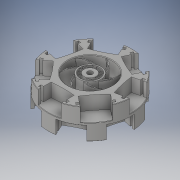
# Autodesk Inventor part: Mecanum Hub
Saved by Autodesk Inventor 2018 (Build 220112000, 112)
## iProperties
Created: 2018-03-28
Part Number: Mecanum Hub
Material: Generic
Document SubType Name: Modeling
Designer: Ajith Thomas
Density: 1 g/cm^3
Appearance: Default
Author: Ajith Thomas
Autodesk Inventor part; units mm, degrees
ref_plane "YZ Plane" through (0, 0, 0) normal (1, 0, 0) x (0, 1, 0)
ref_plane "XZ Plane" through (0, 0, 0) normal (0, 1, 0) x (-1, 0, 0)
ref_plane "XY Plane" through (0, 0, 0) normal (0, 0, 1) x (1, 0, 0)
sketch "Sketch1" plane through (0, 0, 0) normal (0, 1, 0) x (-1, 0, 0)
  circle A0 centre (0, 0) radius 18.5
  circle A1 centre (0, 0) radius 17
  dimension "d0" = 37
  dimension "d1" = 34
  constraints: 2 centre point, 2 coincident
  measures "d0" diameter of A0
  measures "d1" diameter of A1
extrude "Extrusion1" add sketch "Sketch1" along normal mid plane 23
sketch "Sketch2" plane through (0, 11.5, 0) normal (0, 1, 0) x (1, 0, 0)
  circle A0 centre (0, 0) radius 4.75
  circle A1 centre (0, 0) radius 2
  dimension "d4" = 9.5
  dimension "d5" = 4
  constraints: 2 centre point, 2 coincident
  measures "d4" diameter of A0
  measures "d5" diameter of A1
extrude "Extrusion2" add sketch "Sketch2" against normal blind 23
sketch "Sketch3" plane through (0, 0, 0) normal (0, 1, 0) x (-1, 0, 0)
  circle A0 centre (0, 0) radius 17 construction
  circle A1 centre (0, 0) radius 4.75 construction
  line L0 (12.1062, 11.9349) -> (16.389, -4.5168) construction
  arc A2 (4.7443, -0.2334) -> (12.1062, 11.9349) centre (2.5017, 9.4346) ccw
  arc A3 (2.2794, -4.1674) -> (12.1062, 11.9349) centre (0.83, 7.7668) ccw
  arc A4 (2.5742, 3.992) -> (-4.2828, 16.4517) centre (-6.9197, 6.8838) ccw
  arc A5 (4.7487, -0.1097) -> (-4.2828, 16.4517) centre (-6.3112, 4.6022) ccw
  arc A6 (-2.17, 4.2253) -> (-16.389, 4.5168) centre (-9.4214, -2.5508) ccw
  arc A7 (2.4694, 4.0577) -> (-16.389, 4.5168) centre (-7.1412, -3.1645) ccw
  arc A8 (-4.7443, 0.2334) -> (-12.1062, -11.9349) centre (-2.5017, -9.4346) ccw
  arc A9 (-2.2794, 4.1674) -> (-12.1062, -11.9349) centre (-0.83, -7.7668) ccw
  arc A10 (-2.5742, -3.992) -> (4.2828, -16.4517) centre (6.9197, -6.8838) ccw
  arc A11 (-4.7487, 0.1097) -> (4.2828, -16.4517) centre (6.3112, -4.6022) ccw
  arc A12 (2.17, -4.2253) -> (16.389, -4.5168) centre (9.4214, 2.5508) ccw
  arc A13 (-2.4694, -4.0577) -> (16.389, -4.5168) centre (7.1412, 3.1645) ccw
  arc A14 (2.2794, -4.1674) -> (4.7443, -0.2334) centre (0, 0) ccw
  arc A15 (-2.4694, -4.0577) -> (2.17, -4.2253) centre (0, 0) ccw
  arc A16 (-4.7487, 0.1097) -> (-2.5742, -3.992) centre (0, 0) ccw
  arc A17 (-2.2794, 4.1674) -> (-4.7443, 0.2334) centre (0, 0) ccw
  arc A18 (2.4694, 4.0577) -> (-2.17, 4.2253) centre (0, 0) ccw
  arc A19 (4.7487, -0.1097) -> (2.5742, 3.992) centre (0, 0) ccw
  dimension "d8" = 17
  dimension "d11" = 360
  constraints: 42 point on circle, 18 centre point, 6 concentric, 2 end point, 1 tangent, 43 other
  measures "d8" distance of L0.start L0.end
extrude "Extrusion3" add sketch "Sketch3" along normal mid plane 22
sketch "Sketch4" plane through (0, 11, 0) normal (0, 1, 0) x (1, 0, 0)
  circle A0 centre (0, 0) radius 4.75 projected
  arc A1 (-4.7443, 0.2334) -> (-12.1062, -11.9349) centre (-2.5017, -9.4346) ccw projected
  arc A2 (-2.2794, 4.1674) -> (-12.1062, -11.9349) centre (-0.83, -7.7668) ccw projected
  arc A3 (-4.6916, 0.7427) -> (-12.1429, -5.508) centre (-2.5017, -9.4346) ccw
  arc A4 (-3.1813, 3.5273) -> (-12.1429, -5.508) centre (-0.83, -7.7668) ccw
  arc A5 (-3.1813, 3.5273) -> (-4.6916, 0.7427) centre (0, 0) ccw
  arc A6 (-2.989, -3.6917) -> (-1.3014, -13.2701) centre (6.9197, -6.8838) ccw
  arc A7 (-4.6454, -0.9914) -> (-1.3014, -13.2701) centre (6.3112, -4.6022) ccw
  arc A8 (-4.6454, -0.9914) -> (-2.989, -3.6917) centre (0, 0) ccw
  arc A9 (1.7026, -4.4344) -> (10.8415, -7.7621) centre (9.4214, 2.5508) ccw
  arc A10 (-1.4641, -4.5187) -> (10.8415, -7.7621) centre (7.1412, 3.1645) ccw
  arc A11 (-1.4641, -4.5187) -> (1.7026, -4.4344) centre (0, 0) ccw
  arc A12 (4.6916, -0.7427) -> (12.1429, 5.508) centre (2.5017, 9.4346) ccw
  arc A13 (3.1813, -3.5273) -> (12.1429, 5.508) centre (0.83, 7.7668) ccw
  arc A14 (3.1813, -3.5273) -> (4.6916, -0.7427) centre (0, 0) ccw
  arc A15 (2.989, 3.6917) -> (1.3014, 13.2701) centre (-6.9197, 6.8838) ccw
  arc A16 (4.6454, 0.9914) -> (1.3014, 13.2701) centre (-6.3112, 4.6022) ccw
  arc A17 (4.6454, 0.9914) -> (2.989, 3.6917) centre (0, 0) ccw
  arc A18 (-1.7026, 4.4344) -> (-10.8415, 7.7621) centre (-9.4214, -2.5508) ccw
  arc A19 (1.4641, 4.5187) -> (-10.8415, 7.7621) centre (-7.1412, -3.1645) ccw
  arc A20 (1.4641, 4.5187) -> (-1.7026, 4.4344) centre (0, 0) ccw
  dimension "d17" = 360
  constraints: 38 point on circle, 18 centre point, 55 other
extrude "Extrusion4" cut sketch "Sketch4" against normal blind 7 contours A0 A15 A16 | A12 A13 A0 | A0 A18 A19 | A9 A10 A0 | A6 A7 A0 | A0 A3 A4
mirror "Mirror1" about plane through (0, 0, 0) normal (0, 1, 0) of "Extrusion4"
sketch "Sketch5" plane through (0, 11.5, 0) normal (0, 1, 0) x (1, 0, 0)
  circle A0 centre (0, 0) radius 7.5
  circle A1 centre (0, 0) radius 8.5
  dimension "d21" = 15
  dimension "d22" = 17
  constraints: 2 centre point, 2 coincident
  measures "d21" diameter of A0
  measures "d22" diameter of A1
extrude "Extrusion5" add sketch "Sketch5" against normal blind 23
sketch "Sketch6" plane through (0, 0, 0) normal (0, 0, 1) x (1, 0, 0)
  line L0 (-2, 11.5) -> (2, 11.5) construction
  line L1 (2, -11.5) -> (-2, -11.5) construction
  line L2 (-4.75, 11.5) -> (4.75, 11.5) construction
  line L3 (0, 11.5) -> (0, -11.5) construction
  line L4 (7.5, -11.5) -> (-7.5, -11.5) construction
  line L5 (-17, -11.5) -> (-17, 11.5) projected
  line L6 (-17, 0) -> (-15.5, 0) construction
  line L7 (-15.5, 0) -> (-15.5, 0.45)
  line L8 (-15.5, 0) -> (-15.5, -0.45)
  line L9 (-15.5, -0.45) -> (-16, -0.45)
  line L10 (-15.5, 0.45) -> (-16, 0.45)
  line L11 (-16, 0.45) -> (-17, 11.5)
  line L12 (17, -11.5) -> (-17, -11.5) projected
  line L13 (-16, -0.45) -> (-17, -11.5)
  line L14 (-17, 11.5) -> (-17, -11.5)
  point P0 (0, 0)
  dimension "d25" = 1.5
  dimension "d26" = 0.45
  dimension "d27" = 0.45
  dimension "d28" = 0.5
  constraints: 18 end point, 3 horizontal, 3 midpoint, 3 vertical
  measures "d25" distance of L6.start L6.end
  measures "d26" distance of L6.end L7.end
  measures "d27" distance of L6.end L8.end
  measures "d28" distance of L8.end L9.end
revolve "Revolution1" add sketch "Sketch6" angle 360 about axis through (0, 11.5, 0) along (0, -1, 0)
sketch "Sketch7" plane through (0, 0, 0) normal (0, 1, 0) x (-1, 0, 0)
  circle A0 centre (0, 0) radius 8.0302
  constraints: 1 centre point, 1 coincident
extrude "Extrusion6" add sketch "Sketch7" along normal mid plane 10
sketch "Sketch8" plane through (0, 0.45, 0) normal (0, 1, 0) x (0.9294937, 0, 0.368838)
  arc A0 (2.8124, 8.0213) -> (-9.9416, 13.7342) centre (-7.5637, 1.9499) ccw projected
  arc A1 (8.1309, 13.1962) -> (-6.7661, 13.9452) centre (0, 0) ccw projected
  arc A2 (8.1309, 13.1962) -> (-6.7661, 13.9452) centre (0, 0) ccw projected
  arc A3 (2.8124, 8.0213) -> (-9.9416, 13.7342) centre (-7.5637, 1.9499) ccw projected
  arc A4 (-4.0196, 14.9697) -> (-4.0257, 13.4393) centre (-3.3073, 14.2017) ccw
  arc A5 (-4.0196, 14.9697) -> (-6.7661, 13.9452) centre (0, 0) ccw
  arc A6 (-4.0257, 13.4393) -> (-6.7661, 13.9452) centre (-7.5637, 1.9499) ccw
  arc A7 (-14.974, 4.0038) -> (-13.6516, 3.2333) centre (-13.9527, 4.2366) ccw
  arc A8 (-13.6516, 3.2333) -> (-15.46, 1.113) centre (-5.4705, -5.5754) ccw
  arc A9 (-14.974, 4.0038) -> (-15.46, 1.113) centre (0, 0) ccw
  arc A10 (-10.9544, -10.9659) -> (-9.626, -10.206) centre (-10.6453, -9.9651) ccw
  arc A11 (-9.626, -10.206) -> (-8.6939, -12.8322) centre (2.0932, -7.5253) ccw
  arc A12 (-10.9544, -10.9659) -> (-8.6939, -12.8322) centre (0, 0) ccw
  arc A13 (4.0196, -14.9697) -> (4.0257, -13.4393) centre (3.3073, -14.2017) ccw
  arc A14 (4.0257, -13.4393) -> (6.7661, -13.9452) centre (7.5637, -1.9499) ccw
  arc A15 (4.0196, -14.9697) -> (6.7661, -13.9452) centre (0, 0) ccw
  arc A16 (14.974, -4.0038) -> (13.6516, -3.2333) centre (13.9527, -4.2366) ccw
  arc A17 (13.6516, -3.2333) -> (15.46, -1.113) centre (5.4705, 5.5754) ccw
  arc A18 (14.974, -4.0038) -> (15.46, -1.113) centre (0, 0) ccw
  arc A19 (10.9544, 10.9659) -> (9.626, 10.206) centre (10.6453, 9.9651) ccw
  arc A20 (9.626, 10.206) -> (8.6939, 12.8322) centre (-2.0932, 7.5253) ccw
  arc A21 (10.9544, 10.9659) -> (8.6939, 12.8322) centre (0, 0) ccw
  dimension "d34" = 360
  constraints: 38 point on circle, 18 centre point, 2 concentric, 55 other
extrude "Extrusion7" add sketch "Sketch8" against normal blind 0.9
sketch "Sketch9" plane through (0, 11.5, 0) normal (0, 1, 0) x (1, 0, 0)
  circle A0 centre (0, 0) radius 32.5
  circle A1 centre (0, 0) radius 18.5 projected
  dimension "d38" = 65
  constraints: 1 centre point, 1 coincident
  measures "d38" diameter of A0
extrude "Extrusion8" add sketch "Sketch9" against normal blind 23
chamfer "Chamfer1" distance 0.4 angle 45 2 edges at (17, -11.5, 0) (17, 11.5, 0)
sketch "Sketch10" plane through (0, -11.5, 0) normal (0, -1, 0) x (1, 0, 0)
  line L0 (36.1914, -28) -> (-40.3766, -28) construction
  circle A0 centre (0, 0) radius 2 projected
  circle A1 centre (0, 0) radius 32.5 projected
  line L1 (0, 0) -> (0, -32.5) construction
  line L2 (11, -28) -> (11, -29)
  line L3 (11, -28) -> (11, -27)
  line L4 (11, -29) -> (9, -29)
  line L5 (11, -27) -> (9, -27)
  line L6 (-11, -28) -> (-11, -29)
  line L7 (-11, -28) -> (-11, -27)
  line L8 (-11, -29) -> (-9, -29)
  line L9 (-11, -27) -> (-9, -27)
  line L10 (0, -28) -> (0, -35.25) construction
  line L11 (9, -29) -> (9, -34.75)
  line L12 (9, -27) -> (8.8882, -21.25)
  line L13 (-9, -29) -> (-9, -34.75)
  line L14 (-9, -27) -> (-8.8882, -21.25)
  arc A2 (8.8882, -21.25) -> (-8.8882, -21.25) centre (0, -100) ccw
  arc A3 (-9, -34.75) -> (9, -34.75) centre (0, 46) ccw
  point P0 (-11, -26)
  point P1 (0, -20.75)
  point P2 (0, -35)
  dimension "d45" = 28
  dimension "d48" = 11
  dimension "d49" = 11
  dimension "d50" = 1
  dimension "d51" = 1
  dimension "d52" = 2
  dimension "d53" = 2
  dimension "d54" = 1
  dimension "d58" = 7.25
  dimension "d59" = 7.25
  dimension "d60" = 6.75
  dimension "d61" = 6.75
  dimension "d62" = 35.25
  dimension "d64" = 7
  dimension "d65" = 35
  constraints: 30 end point, 7 symmetric about line, 6 point on circle, 5 point on line, 4 vertical, 3 horizontal, 2 centre point, 1 coincident, 1 vertical alignment, 1 other
  measures "d45" distance from line of point (0, 0) L0
  measures "d48" distance from line of L1 L2.start
  measures "d49" distance from line of L1 point (-11, -26)
  measures "d50" distance of L2.start L2.end
  measures "d51" distance of L2.start L3.end
  measures "d52" distance of L2.end L4.end
  measures "d53" distance of L3.end L5.end
  measures "d54" distance between parallel lines of L0 L4
  measures "d58" distance of L10.start L10.end
  measures "d59" distance from line of L0 point (0, -20.75)
  measures "d60" distance from line of L11.end L0
  measures "d61" distance from line of L12.end L0
  measures "d62" distance of point (0, 0) point (0, -35.25)
  measures "d64" distance from line of L0 point (0, -35)
  measures "d65" distance of point (0, 0) point (0, -35)
extrude "Extrusion9" cut sketch "Sketch10" against normal blind 10.5 contours L13 L8 L6 L7 L9 L14 A2 L12 L5 L3 L2 L4 L11 A1 | A1 L11 A3 L13 picked at (0.9894, -28.5072)
pattern_circular "Circular Pattern1" count 7 over 360 about axis through (0, 11.5, 0) along (0, -1, 0) of "Extrusion9"
sketch "Sketch11" plane through (0, 11.5, 0) normal (0, 1, 0) x (1, 0, 0)
  arc A0 (9, 31.229) -> (-9, 31.229) centre (0, 0) ccw projected
  line L0 (9, 29) -> (9, 31.229) projected
  line L1 (11, 29) -> (9, 29) projected
  line L2 (11, 27) -> (11, 29) projected
  line L3 (9, 27) -> (11, 27) projected
  line L4 (8.8882, 21.25) -> (9, 27) construction
  arc A1 (-8.8882, 21.25) -> (8.8882, 21.25) centre (0, 100) ccw construction
  line L5 (-9, 27) -> (-8.8882, 21.25) projected
  line L6 (-11, 27) -> (-9, 27) projected
  line L7 (-11, 29) -> (-11, 27) projected
  line L8 (-9, 29) -> (-11, 29) projected
  line L9 (-9, 31.229) -> (-9, 29) projected
  arc A2 (-9, 31.229) -> (-18.8044, 26.5074) centre (0, 0) ccw projected
  arc A3 (18.8044, 26.5074) -> (9, 31.229) centre (0, 0) ccw projected
  arc A4 (-9, 31.229) -> (-18.8044, 26.5074) centre (0, 0) ccw
  circle A5 centre (0, 0) radius 32.5 projected
  arc A6 (18.8044, 26.5074) -> (9, 31.229) centre (0, 0) ccw
  arc A7 (-18.8044, 26.5074) -> (-30.0272, 12.4345) centre (0, 0) ccw projected
  line L10 (-9, 31.229) -> (-9, 29) projected
  line L11 (-21.6567, 24.233) -> (-20.6897, 22.2247)
  line L12 (-11, 29) -> (-11, 27) projected
  line L13 (-20.6897, 22.2247) -> (-22.4917, 21.3571)
  line L14 (-22.4917, 21.3571) -> (-21.6241, 19.5551)
  line L15 (-21.6241, 19.5551) -> (-19.8221, 20.4227)
  line L16 (-9, 27) -> (-8.8882, 21.25) projected
  line L17 (-19.8221, 20.4227) -> (-17.2269, 15.2904)
  line L18 (9, 29) -> (9, 31.229) projected
  line L19 (11, 29) -> (9, 29) projected
  line L20 (-5.4386, 32.0417) -> (-4.4717, 30.0334)
  line L21 (11, 27) -> (11, 29) projected
  line L22 (-4.4717, 30.0334) -> (-2.6697, 30.901)
  line L23 (-2.6697, 30.901) -> (-1.802, 29.099)
  line L24 (8.8882, 21.25) -> (9, 27) projected
  line L25 (-1.802, 29.099) -> (-3.604, 28.2314)
  line L26 (-3.604, 28.2314) -> (-1.2103, 23.0021)
  arc A8 (-8.8882, 21.25) -> (8.8882, 21.25) centre (0, 100) ccw projected
  arc A9 (-17.2269, 15.2904) -> (-1.2103, 23.0021) centre (-43.3816, 90.1001) ccw
  arc A10 (-5.4386, 32.0417) -> (-21.6567, 24.233) centre (0, 0) ccw
  line L27 (0, 0) -> (-14.1012, 29.2815) construction
  line L28 (0, 32.5) -> (0, 0) construction
  dimension "d71" = 25.714
  constraints: 24 end point, 9 point on circle, 5 perpendicular, 4 centre point, 1 concentric, 1 vertical, 4 other
  measures "d71" angle of L28 L27
extrude "Extrusion10" cut sketch "Sketch11" against normal blind 10.5 contours L20 L22 L23 L25 L26 A9 A8 L5 L6 L7 L8 L9 A0 | L9 L8 L7 L6 L5 A8 A9 L17 L15 L14 L13 L11 A5 A2
pattern_circular "Circular Pattern2" count 7 over 360 about axis through (0, 11.5, 0) along (0, -1, 0) of "Extrusion10"
fillet "Fillet2" radius 0.3 27 edges at (14.099, 11.5, 29.2825) (31.6846, 11.5, 7.2343) (25.411, 11.5, -20.2615) (0.0024, 11.5, -32.5) (-25.408, 11.5, -20.2653) (-31.6857, 11.5, 7.2296) (-14.1034, 11.5, 29.2804) (0, -11.5, 32.5) (-25.4095, -11.5, 20.2634) (-31.6852, -11.5, -7.2319) (-14.1012, -11.5, -29.2815) (14.1012, -11.5, -29.2815) (31.6852, -11.5, -7.2319) (25.4095, -11.5, 20.2634) (14.1012, -1, 29.2815) (-0.0024, 1, 32.5) (-14.1012, -1, 29.2815) (25.408, 1, 20.2653) (-25.411, 1, 20.2615) (-31.6852, -1, 7.2319) (-25.4095, -1, -20.2634) (-14.099, 1, -29.2825) (0, -1, -32.5) (14.1034, 1, -29.2804) (32.4871, 1, 0.9142) (31.4698, 1, -8.118) (25.4095, -1, -20.2634)
sketch "Sketch12" plane through (0, 11.5, 0) normal (0, 1, 0) x (1, 0, 0)
  circle A0 centre (0, 0) radius 2 projected
extrude "Extrusion11" cut sketch "Sketch12" against normal blind 62.3875
body "Solid1"
